Handrail (Autodesk Fusion 360 design; units mm, degrees)
Autodesk Fusion 360 part; units mm, degrees
sketch "Sketch1" plane through (0, 0, 0) normal (0, 0, 1) x (1, 0, 0)
  line L0 (0, 150) -> (50, 150)
  line L1 (50, 150) -> (50, 0)
  line L2 (50, 0) -> (0, 0)
  line L3 (0, 0) -> (0, 150)
  line L4 (0, 80) -> (-50, 80)
  line L5 (-50, 80) -> (-50, 30)
  line L6 (-50, 30) -> (0, 30)
  line L7 (0, 30) -> (0, 80)
  line L8 (-25, 30) -> (-27.6047, 44.7721)
  line L9 (-27.6047, 44.7721) -> (-40.4072, 42.5147)
  line L10 (-40.4072, 42.5147) -> (-37.8025, 27.7426)
  line L11 (-37.8025, 27.7426) -> (-25, 30)
  dimension "d1" = 50
  dimension "d2" = 150
  dimension "d3" = 30
  dimension "d4" = 50
  dimension "d5" = 50
  dimension "d8" = 13
  dimension "d9" = 15
  dimension "d10" = 100
  constraint horizontal L0
  constraint vertical L1
  constraint horizontal L2
  constraint vertical L3
  constraint coincident L2.end L3.start
  constraint horizontal L4
  constraint vertical L5
  constraint horizontal L6
  constraint vertical L7
  constraint coincident L3 L4.start
  constraint perpendicular L8 L9
  constraint parallel L8 L10
  constraint parallel L9 L11
  constraint midpoint L6 L8.start
  measures "d1" distance of L0.start L0.end
  measures "d2" distance of L0.start L2.end
  measures "d3" distance of L2.end L6.end
  measures "d4" distance of L4.start L4.end
  measures "d5" distance of L4.end L5.end
  measures "d8" distance of L8.start L10.end
  measures "d9" distance of L9.end L10.end
  measures "d10" angle of L6 L8
extrude "Extrude1" add sketch "Sketch1" along normal blind 3000 contours L0 L1 L2 L3 L7 makes body 1
extrude "Extrude2" add sketch "Sketch1" along normal blind 2750 from surface at 150 separate body contours L3 L4 L5 L6 L7 L8 L9 L10 makes body 2
fillet "Fillet1" radius 10 2 edges at (50, 150, 1500) (0, 150, 1500) on bodies 1
sketch "Sketch2" plane through (0, 0, 0) normal (0, 0, 1) x (1, 0, 0)
  line L0 (-50, -1913.7171) -> (-250, -1913.7171)
  line L1 (-250, -1913.7171) -> (-250, 2086.2829)
  line L2 (-250, 2086.2829) -> (-50, 2086.2829)
  line L3 (-50, 2086.2829) -> (-50, -1913.7171)
  line L4 (-50, 80) -> (-50, 30)
  dimension "d17" = 200
  dimension "d18" = 4000
  constraint horizontal L0
  constraint vertical L1
  constraint horizontal L2
  constraint vertical L3
  constraint collinear L3 L4
  measures "d17" distance of L1.end L2.end
  measures "d18" distance of L0.end L1.end
extrude "Extrude3" add sketch "Sketch2" along normal blind 5000 from surface at -1000 separate body makes body 3
move_body "Move1" bodies 1 2 to x (1, 0, 0) y (0, 0.906308, -0.422618) z (0, 0.422618, 0.906308) at (0, -481.1251, 128.9171)
ref_plane "WorkPlane1" through (-150, 86.2829, 2780) normal (0, 0, 1) x (1, 0, 0)
split "Split1" by plane through (-150, 86.2829, 2780) normal (0, 0, 1) bodies 1 makes body 4 at (16.6667, 829.0241, 2828.1183)
ref_plane "WorkPlane2" through (-150, 86.2829, 140) normal (0, 0, -1) x (-1, 0, 0)
split "Split2" by plane through (-150, 86.2829, 140) normal (0, 0, -1) bodies 1 makes body 5 at (16.6667, -438.8307, 109.1949)
hidden bodies 4 5
